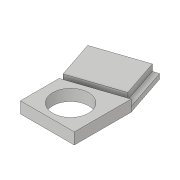
# Autodesk Inventor part: Lidar Sensor Case Piece 2
Saved by Autodesk Inventor 2018.3 (Build 223284000, 284)
## iProperties
Created: 2019-02-26
Part Number: Lidar Sensor Case Piece 2
Material: Generic
Document SubType Name: Modeling
Designer: aye06091
Mass: 5.17749 g
Surface Area: 32.7073 cm^2
Volume: 5.17749 cm^3
Density: 1 g/cm^3
Appearance: Default
Author: aye06091
Autodesk Inventor part; units mm, degrees
ref_plane "YZ Plane" through (0, 0, 0) normal (1, 0, 0) x (0, 1, 0)
ref_plane "XZ Plane" through (0, 0, 0) normal (0, 1, 0) x (-1, 0, 0)
ref_plane "XY Plane" through (0, 0, 0) normal (0, 0, 1) x (1, 0, 0)
sketch "Sketch1" plane through (0, 0, 0) normal (0, 1, 0) x (-1, 0, 0)
  line L0 (-8.0312, -19.6194) -> (-8.0312, -0.5694)
  line L1 (-8.0312, -0.5694) -> (-34.5277, -0.5694)
  line L2 (-34.5277, -0.5694) -> (-34.5277, -28.5056)
  line L3 (18.6455, 5.0782) -> (18.6456, 5.0782)
  line L4 (-1.974, -37.6808) -> (-8.0312, -19.6194)
  line L5 (-34.5277, -28.5056) -> (-27.4611, -49.5771)
  line L6 (-1.974, -37.6808) -> (-0.9645, -40.691)
  line L7 (-27.4611, -49.5771) -> (-0.9645, -40.691)
  circle A0 centre (-21.2795, -12.0217) radius 8.7948
  line L8 (-8.0312, -0.5694) -> (-8.0312, -19.6194)
  line L9 (-8.0312, -19.6194) -> (-0.9645, -40.691)
  line L10 (-0.9645, -40.691) -> (-27.4611, -49.5771)
  line L11 (-27.4611, -49.5771) -> (-34.5277, -28.5056)
  line L12 (-34.5277, -28.5056) -> (-34.5277, -0.5694)
  line L13 (-34.5277, -0.5694) -> (-8.0312, -0.5694)
  point P0 (0, 0)
  dimension "d0" = 19.05
  dimension "d1" = 22.225
  dimension "d2" = 27.9469
  dimension "d3" = 26.4965
  dimension "d4" = 17.5895
  dimension "d20" = 11.4522
  dimension "d21" = 13.2483
  constraints: 28 end point, 3 perpendicular, 2 parallel, 1 centre point, 1 collinear, 1 vertical
  measures "d0" distance of L0.start L0.end
  measures "d1" distance of L4.end L6.end
  measures "d2" distance of L5.end L7.end
  measures "d3" distance of L0.end L1.end
  measures "d4" diameter of A0
  measures "d20" distance from line of L1 A0.centre
  measures "d21" distance from line of L0 A0.centre
extrude "Extrusion1" add sketch "Sketch1" along normal blind 5.6134
sketch "Sketch2" plane through (0, 5.6134, 0) normal (0, 1, 0) x (1, 0, 0)
  line L0 (34.5277, 28.5056) -> (8.0312, 19.6194)
  line L1 (8.0312, 19.6194) -> (7.0701, 22.4851)
  line L2 (7.0701, 22.4851) -> (33.5666, 31.3713)
  line L3 (31.5176, 27.4961) -> (29.9884, 26.9832)
  line L4 (34.5277, 28.5056) -> (27.4611, 49.5771) projected
  point P0 (0, 0)
  point P1 (0, 0)
  dimension "d11" = 3.0226
  constraints: 8 end point, 4 point on line, 1 parallel, 1 perpendicular
  measures "d11" distance between parallel lines of L2 L0
extrude "Extrusion2" cut sketch "Sketch2" against normal blind 3.175
sketch "Sketch3" plane through (0, 5.6134, 0) normal (0, 1, 0) x (1, 0, 0)
  line L0 (7.0701, 22.4852) -> (33.5666, 31.3713) projected
  line L1 (33.5666, 31.3713) -> (27.4611, 49.5771) projected
  line L2 (27.4611, 49.5771) -> (0.9645, 40.691) projected
  line L3 (24.8, 48.6846) -> (30.9056, 30.4789)
  point P0 (0, 0)
  dimension "d17" = 2.8067
  constraints: 2 end point, 2 point on line, 1 parallel
  measures "d17" distance between parallel lines of L1 L3
extrude "Extrusion3" cut sketch "Sketch3" against normal blind 3.175
body "Solid1"
